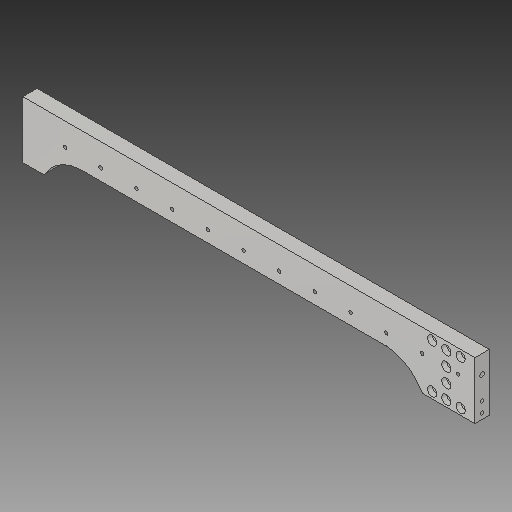
# Autodesk Inventor part: Xcolum
Saved by Autodesk Inventor 2019 (Build 230136000, 136)
## iProperties
Created: 2018-10-03
Part Number: Xcolum
Material: Aluminum 6061-AHC
Document SubType Name: Modeling
Designer: LillaHunden
Mass: 228.044 g
Surface Area: 268.68 cm^2
Volume: 84.4607 cm^3
Density: 2.7 g/cm^3
Appearance: Aluminum - Dark
Author: LillaHunden
Autodesk Inventor part; units mm, degrees
ref_plane "YZ Plane" through (0, 0, 0) normal (1, 0, 0) x (0, 1, 0)
ref_plane "XZ Plane" through (0, 0, 0) normal (0, 1, 0) x (-1, 0, 0)
ref_plane "XY Plane" through (0, 0, 0) normal (0, 0, 1) x (1, 0, 0)
sketch "Sketch1" plane through (0, 0, 0) normal (0, 0, 1) x (1, 0, 0)
  line L0 (-16.5, -29.1453) -> (300, -29.1453)
  line L1 (300, -29.1453) -> (300, 10.8547)
  line L2 (300, 10.8547) -> (-16.5, 10.8547)
  line L3 (-16.5, 10.8547) -> (-16.5, -29.1453)
  line L4 (-14.5, -10.6453) -> (-14.5, 0.3547) construction
  point P0 (0, 0)
  dimension "d1" = 40
  dimension "d29" = 2
  constraints: 8 end point, 2 parallel, 1 horizontal, 1 perpendicular
  measures "d1" distance of L1.end L0.end
  measures "d29" distance between parallel lines of L4 L3
extrude "Extrusion1" add sketch "Sketch1" along normal blind 10
sketch "Sketch2" plane through (300, -29.1453, 0) normal (1, 0, 0) x (0, 0, -1)
  point P0 (-5, 3.8516)
  point P1 (-5, 11.1484)
  point P2 (4.1697, 3.85)
  point P3 (4.1697, 11.15)
hole "Hole1" at (300, -25.2937, 5) at (300, -17.9969, 5) at (300, -25.2953, -4.1697) at (300, -17.9953, -4.1697) direction (-1, 0, 0) diameter 2.459 depth 10.4 tip angle 120 thread size "M3x0.5" class "6H" standard "ISO Metric profile"
sketch "Sketch3" plane through (0, 0, 10) normal (0, 0, 1) x (1, 0, 0)
  line L0 (-16.5, -29.1453) -> (300, -29.1453) projected
  arc A0 (262.975, -29.1453) -> (237.975, -13.1453) centre (236.4208, -43.105) ccw
  line L1 (237.975, -13.1453) -> (23.5, -13.1453)
  line L2 (-16.5, -29.1453) -> (-1.5, -29.1453)
  arc A1 (23.5, -13.1453) -> (-1.5, -29.1453) centre (25.0542, -43.105) ccw
  circle A2 centre (290, -44.6453) radius 3.25 construction
  circle A3 centre (270, -44.6453) radius 3.25 construction
  circle A4 centre (270, 26.3547) radius 3.25 construction
  line L3 (300, -54.1453) -> (300, 35.8547) construction
  line L4 (300, 35.8547) -> (262.975, 35.8547) construction
  line L5 (262.975, 35.8547) -> (262.975, -54.1453) construction
  line L6 (262.975, -54.1453) -> (300, -54.1453) construction
  circle A5 centre (290, 26.3547) radius 3.25 projected
  circle A6 centre (266.0501, -14.92) radius 1.621 projected
  circle A7 centre (265, 1.4718) radius 1.621 projected
  circle A8 centre (290, 1.4718) radius 1.621 projected
  circle A9 centre (270, 6.3547) radius 1.2295 projected
  circle A10 centre (270, -24.6453) radius 1.2295 projected
  circle A11 centre (290, -24.6453) radius 1.2295 projected
  circle A12 centre (290, 6.3547) radius 1.2295 projected
  circle A13 centre (280, -4.6453) radius 1.2295 projected
  circle A14 centre (280, -24.6453) radius 1.2295 projected
  circle A15 centre (280, -14.6453) radius 1.2295 projected
  circle A16 centre (280, 5.3547) radius 1.2295 projected
  point P0 (0, 0)
  point P1 (292.0748, -22.1438)
  point P2 (290.1996, -21.4014)
  dimension "d12" = 30
  dimension "d16" = 15
  dimension "d17" = 30
  dimension "d18" = 25
  dimension "d19" = 25
  dimension "d20" = 16
  constraints: 4 end point, 4 point on circle, 3 point on line, 2 centre point, 1 horizontal, 1 other
  measures "d12" radius of A0
  measures "d16" distance of L0.start L2.end
  measures "d17" radius of A1
  measures "d18" horizontal distance of A0.start L1.start
  measures "d19" horizontal distance of L2.end L1.end
  measures "d20" distance between parallel lines of L0 L1
extrude "Extrusion2" cut sketch "Sketch3" against normal through all contours A1 L1 A0 L0
fillet "Fillet1" radius 2 2 edges at (-1.5, -29.1453, 5) (262.975, -29.1453, 5)
sketch "Sketch4" plane through (0, 0, 10) normal (0, 0, 1) x (1, 0, 0)
  point P0 (288, -5.1453)
  point P1 (263, -5.1453)
  point P2 (238, -5.1453)
  point P3 (213, -5.1453)
  point P4 (188, -5.1453)
  point P5 (163, -5.1453)
  point P6 (88, -5.1453)
  point P7 (63, -5.1453)
  point P8 (38, -5.1453)
  point P9 (13, -5.1453)
  point P10 (138, -5.1453)
  point P11 (113, -5.1453)
hole "Hole3" at (288, -5.1453, 10) at (263, -5.1453, 10) at (238, -5.1453, 10) at (213, -5.1453, 10) at (188, -5.1453, 10) at (163, -5.1453, 10) at (88, -5.1453, 10) at (63, -5.1453, 10) at (38, -5.1453, 10) at (13, -5.1453, 10) at (138, -5.1453, 10) at (113, -5.1453, 10) direction (0, 0, -1) diameter 2.459 depth 11 tip angle 120 thread size "M3x0.5" class "6H" standard "ISO Metric profile"
sketch "Sketch5" plane through (300, -29.1453, 0) normal (1, 0, 0) x (0, 0, -1)
  point P0 (-5, 27.2319)
  point P1 (4.1697, 27.2319)
  point P2 (4.1697, 43.2319)
  point P3 (4.1697, 59.2319)
  point P4 (4.1697, -12.7681)
hole "Hole5" at (300, -1.9134, 5) at (300, -1.9134, -4.1697) at (300, 14.0866, -4.1697) at (300, 30.0866, -4.1697) at (300, -41.9134, -4.1697) direction (-1, 0, 0) diameter 3.242 depth 10.5 tip angle 120 thread size "M4x0.7" class "6H" standard "ISO Metric profile"
sketch "Sketch6" plane through (0, 0, 10) normal (0, 0, 1) x (1, 0, 0)
  line L0 (300, -20.4469) -> (300, -15.5469) construction
  line L1 (300, -28.0437) -> (300, -22.5437) construction
  line L2 (300, -4.1634) -> (300, 0.3366) construction
  circle A0 centre (290, 26.3547) radius 3.25 construction
  circle A1 centre (290, -44.6453) radius 3.25 construction
  circle A2 centre (270, -44.6453) radius 3.25 construction
  circle A3 centre (270, 26.3547) radius 3.25 construction
  line L3 (300, -54.1453) -> (300, 35.8547) construction
  line L4 (300, 35.8547) -> (262.975, 35.8547) construction
  line L5 (262.975, 35.8547) -> (262.975, -54.1453) construction
  line L6 (262.975, -54.1453) -> (300, -54.1453) construction
  circle A4 centre (270, 6.3547) radius 1.2295 projected
  circle A5 centre (270, -24.6453) radius 1.2295 projected
  circle A6 centre (290, -24.6453) radius 1.2295 projected
  circle A7 centre (290, 6.3547) radius 1.2295 projected
  line L7 (290, -24.6453) -> (270, -24.6453) construction
  circle A8 centre (280, -4.6453) radius 1.2295 projected
  circle A9 centre (280, -24.6453) radius 1.2295 projected
  circle A10 centre (280, -14.6453) radius 1.2295 projected
  circle A11 centre (280, 5.3547) radius 1.2295 projected
  point P0 (0, 0)
  point P1 (280, -24.6453)
  point P2 (280, -14.6453)
  point P3 (280, -4.6453)
  point P4 (280, 5.3547)
  point P5 (280, -24.6453)
  dimension "d68" = 10
  dimension "d69" = 10
  dimension "d70" = 10
  constraints: 3 vertical alignment, 2 end point, 1 coincident, 1 horizontal, 1 horizontal alignment, 1 midpoint
  measures "d68" distance of point (280, -14.645) point (280, -24.645)
  measures "d69" distance of point (280, -4.645) point (280, -14.645)
  measures "d70" distance of point (280, -4.645) point (280, 5.355)
sketch "Sketch9" plane through (0, 0, 10) normal (0, 0, 1) x (1, 0, 0)
  point P0 (270, -24.6453)
  point P1 (290, -24.6453)
  point P2 (270, 6.3547)
  point P3 (290, 6.3547)
hole "Hole10" at (270, -24.6453, 10) at (290, -24.6453, 10) at (270, 6.3547, 10) at (290, 6.3547, 10) direction (0, 0, -1) diameter 3.2 depth 10 counterbore diameter 6.5 counterbore depth 3.4
sketch "Sketch10" plane through (0, 0, 10) normal (0, 0, 1) x (1, 0, 0)
  point P0 (280, -24.6453)
  point P1 (280, -14.6453)
  point P2 (280, -4.6453)
  point P3 (280, 5.3547)
hole "Hole12" at (280, -24.6453, 10) at (280, -14.6453, 10) at (280, -4.6453, 10) at (280, 5.3547, 10) direction (0, 0, -1) diameter 3.2 depth 10 counterbore diameter 6.5 counterbore depth 3.4
sketch "Sketch12" plane through (-16.5, -29.1453, 0) normal (-1, 0, 0) x (0, 0, 1)
  point P0 (5, 8)
  point P1 (5, 16)
  point P2 (5, 24)
  point P3 (5, 32)
hole "Hole15" at (-16.5, -21.1453, 5) at (-16.5, -13.1453, 5) at (-16.5, -5.1453, 5) at (-16.5, 2.8547, 5) direction (1, 0, 0) diameter 2.459 depth 8.4 tip angle 120 thread size "M3x0.5" class "6H" standard "ISO Metric profile"
equation "\"d12\" = d11"
equation "\"d17\" = d12"
equation "\"d19\" = d18"
equation "\"d11\" = 30"
body "Solid1"
